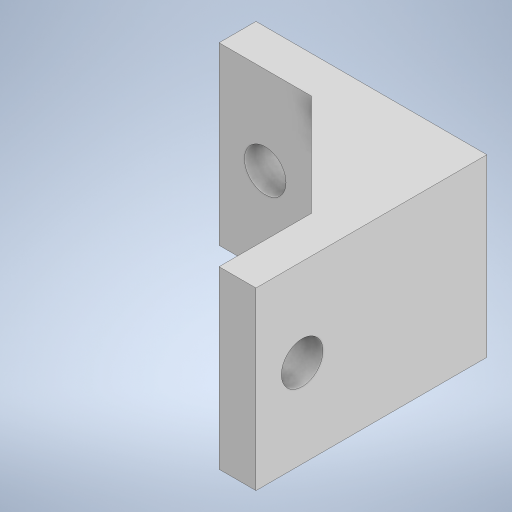
# Autodesk Inventor part: KeNhom40
Saved by Autodesk Inventor 2023 (Build 270158000, 158)
## iProperties
Created: 2025-04-01
Part Number: KeNhom40
Material: Generic
Document SubType Name: Modeling
Designer: huyqu
Density: 1 g/cm^3
Appearance: Default
Author: huyqu
Autodesk Inventor part; units mm, degrees
ref_plane "YZ Plane" through (0, 0, 0) normal (1, 0, 0) x (0, 1, 0)
ref_plane "XZ Plane" through (0, 0, 0) normal (0, 1, 0) x (-1, 0, 0)
ref_plane "XY Plane" through (0, 0, 0) normal (0, 0, 1) x (1, 0, 0)
sketch "Sketch1" plane through (0, 0, 0) normal (0, 0, 1) x (1, 0, 0)
  line L0 (0, 0) -> (50, 0)
  line L1 (50, 0) -> (50, 38)
  line L2 (50, 38) -> (0, 38)
  line L3 (0, 38) -> (0, 0)
  dimension "d0" = 38
  dimension "d3" = 50
  constraints: 8 end point, 2 parallel, 1 horizontal, 1 perpendicular
  measures "d0" distance between parallel lines of L0 L2
  measures "d3" distance of L1.end L2.end
extrude "Extrusion1" add sketch "Sketch1" along normal blind 8
sketch "Sketch2" plane through (0, 0, 8) normal (0, 0, 1) x (1, 0, 0)
  line L0 (50, 0) -> (50, 38) projected
  line L1 (0, 0) -> (50, 0) projected
  line L2 (50, 38) -> (42, 38)
  line L3 (42, 38) -> (42, 0)
  line L4 (42, 0) -> (50, 0)
  line L5 (50, 0) -> (50, 38)
  dimension "d4" = 8
  constraints: 8 end point, 2 parallel, 1 horizontal, 1 perpendicular, 1 point on line
  measures "d4" distance between parallel lines of L0 L3
extrude "Extrusion2" add sketch "Sketch2" along normal blind 42
sketch "Sketch3" plane through (0, 0, 0) normal (0, -1, 0) x (1, 0, 0)
  line L0 (42, 8) -> (42, 50) projected
  line L1 (42, 30) -> (20, 8)
  line L2 (0, 8) -> (42, 8) projected
  line L3 (0, 0) -> (50, 0) projected
  line L4 (50, 0) -> (50, 50) projected
  dimension "d7" = 30
  dimension "d8" = 30
  constraints: 2 end point, 2 point on line
  measures "d7" distance from line of L3 L1.start
  measures "d8" distance from line of L4 L1.end
extrude "Extrusion3" add sketch "Sketch3" against normal up to surface (38 mm away)
sketch "Sketch4" plane through (42, 0, 50) normal (-1, 0, 0) x (0, 0, 1)
  circle A0 centre (-10, 19) radius 4.5
  line L0 (0, 38) -> (0, 0) projected
  line L1 (-20, 38) -> (0, 38) projected
  point P0 (-50, 0)
  dimension "d11" = 10
  dimension "d12" = 19
  dimension "d13" = 9
  constraints: 1 centre point
  measures "d11" distance from line of A0.centre L0
  measures "d12" distance from line of A0.centre L1
  measures "d13" diameter of A0
extrude "Extrusion4" cut sketch "Sketch4" against normal through all
sketch "Sketch5" plane through (0, 0, 8) normal (0, 0, 1) x (1, 0, 0)
  circle A0 centre (10, 19) radius 4.5
  line L0 (0, 38) -> (0, 0) projected
  line L1 (0, 0) -> (20, 0) projected
  dimension "d16" = 10
  dimension "d17" = 19
  dimension "d18" = 9
  constraints: 1 centre point
  measures "d16" distance from line of L0 A0.centre
  measures "d17" distance from line of A0.centre L1
  measures "d18" diameter of A0
extrude "Extrusion5" cut sketch "Sketch5" against normal blind 10
body "Solid1"
